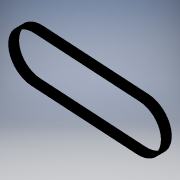
# Autodesk Inventor part: Belt
Saved by Autodesk Inventor 2018 (Build 220112000, 112)
## iProperties
Created: 2018-01-26
Part Number: Belt
Material: Generic
Document SubType Name: Modeling
Designer: Apple
Density: 1 g/cm^3
Appearance: Default
Author: Apple
Autodesk Inventor part; units mm, degrees
ref_plane "YZ Plane" through (0, 0, 0) normal (1, 0, 0) x (0, 1, 0)
ref_plane "XZ Plane" through (0, 0, 0) normal (0, 1, 0) x (-1, 0, 0)
ref_plane "XY Plane" through (0, 0, 0) normal (0, 0, 1) x (1, 0, 0)
sketch "Sketch1" plane through (0, 0, 0) normal (0, 0, 1) x (1, 0, 0)
  circle A0 centre (-32.198, -0.1238) radius 50.8 projected
  circle A1 centre (123.0816, -9.7192) radius 50.8 projected
  arc A2 (-30.1614, 32.8334) -> (-34.2345, -33.0809) centre (-32.198, -0.1238) ccw
  arc A3 (121.045, -42.6763) -> (125.1181, 23.238) centre (123.0816, -9.7192) ccw
  line L0 (121.045, -42.6763) -> (-34.2345, -33.0809)
  line L1 (125.1181, 23.238) -> (-30.1614, 32.8334)
  arc A4 (120.8492, -45.8453) -> (125.314, 26.4069) centre (123.0816, -9.7192) ccw
  line L2 (120.8492, -45.8453) -> (-34.4304, -36.2499)
  arc A5 (-29.9656, 36.0023) -> (-34.4304, -36.2499) centre (-32.198, -0.1238) ccw
  line L3 (-29.9656, 36.0023) -> (125.314, 26.4069)
  point P0 (0, 0)
  dimension "d0" = 66.04
  dimension "d1" = 66.04
  dimension "d2" = 3.175
  constraints: 8 end point, 8 point on circle, 4 centre point, 2 coincident, 2 parallel, 2 tangent, 3 other
  measures "d0" diameter of A2
  measures "d1" diameter of A3
  measures "d2" radial gap between concentric circles of A3 A4
extrude "Extrusion1" add sketch "Sketch1" along normal mid plane 12.7 contours L1 A2 L0 A0 L2 A5 L3 | A0 L3 A1 L1 | L0 A1 L2 A0 | A1 L3 A4 L2 L0 A3 L1
body "Solid1"
